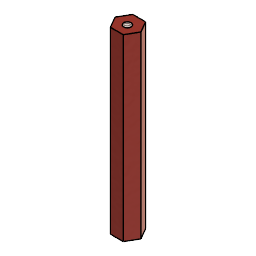
second_pillar (Autodesk Fusion 360 design; units mm, degrees)
part number: 2026-06-29-20-18-54-859
Autodesk Fusion 360 part; units mm, degrees
sketch "Sketch1" plane through (0, 0, 0) normal (0, 0, 1) x (1, 0, 0)
  line L0 (32.8868, 25) -> (35.7735, 30)
  line L1 (35.7735, 30) -> (32.8868, 35)
  line L2 (32.8868, 35) -> (27.1132, 35)
  line L3 (27.1132, 35) -> (24.2265, 30)
  line L4 (24.2265, 30) -> (27.1132, 25)
  line L5 (27.1132, 25) -> (32.8868, 25)
  point P0 (30, 30)
  dimension "d1" = 5
  measures "d1" distance of P0 L5
extrude "Extrude1" add sketch "Sketch1" along normal blind 80
hole "Hole1" at (29.7914, 30.1949, 0) direction (0, 0, 1) diameter 3.332 depth 6 tip angle 180
thread "Thread1" "ISO Metric profile 4.0 M4x0.7 M4x0.7 6H" thread offset 0 thread depth 7.4
hole "Hole2" at (30, 29.7466, 80) direction (0, 0, -1) diameter 3.332 depth 6 tip angle 180
thread "Thread3" "ISO Metric profile 4.0 M4x0.7 M4x0.7 6H" thread offset 0 thread depth 7.4
